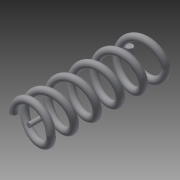
# Autodesk Inventor part: Spring
Saved by Autodesk Inventor 2015 (Build 190159000, 159)
## iProperties
Created: 2017-01-08
Part Number: Spring
Material: Generic
Document SubType Name: Modeling
Designer: Ernest
Density: 1 g/cm^3
Appearance: Default
Mass: 0.268639 g
Surface Area: 7.30223 cm^2
Volume: 0.268639 cm^3
Author: Ernest
Autodesk Inventor part; units mm, degrees
ref_plane "YZ Plane" through (0, 0, 0) normal (1, 0, 0) x (0, 1, 0)
ref_plane "XZ Plane" through (0, 0, 0) normal (0, 1, 0) x (-1, 0, 0)
ref_plane "XY Plane" through (0, 0, 0) normal (0, 0, 1) x (1, 0, 0)
sketch "Sketch1" plane through (0, 0, 0) normal (0, 0, 1) x (1, 0, 0)
  line L0 (0, 0) -> (0, 25)
  circle A0 centre (4, 0) radius 0.75
  dimension "d0" = 25
  dimension "d1" = 1.5
  dimension "d2" = 4
  constraints: 2 end point, 1 centre point, 1 vertical
  measures "d0" distance of L0.start L0.end
  measures "d1" diameter of A0
  measures "d2" distance of L0.start A0.centre
coil "Coil1" sketch "Sketch1" operation add axis through (0, 0, 0) along (0, 1, 0) pitch 5 turns 5 hand right
sketch "Sketch2" plane through (4, 0, 0) normal (0, 0, 1) x (1, 0, 0)
  circle A0 centre (0, 0) radius 0.75
  line L0 (-4, 0) -> (-4, -1.8881)
  constraints: 2 end point, 1 centre point, 1 vertical
revolve "Revolution1" add sketch "Sketch2" angle 180 about axis through (0, 0, 0) along (0, -1, 0)
sketch "Sketch3" plane through (4, 25, 0) normal (0, 0, -1) x (-1, 0, 0)
  circle A0 centre (0, 0) radius 0.75 projected
  line L0 (4, 0) -> (4, 3.1706)
  point P0 (4, -25)
  point P1 (-0.75, 0)
  constraints: 2 end point, 1 horizontal alignment, 1 vertical
revolve "Revolution2" add sketch "Sketch3" angle 180 about axis through (0, 25, 0) along (0, 1, 0)
sketch "Sketch4" plane through (0, 0, 0) normal (0, 1, 0) x (-1, 0, 0)
  circle A0 centre (0, 0) radius 0.5
  dimension "d13" = 1
  constraints: 1 centre point, 1 coincident
  measures "d13" diameter of A0
extrude "Extrusion1" add sketch "Sketch4" along normal blind 2 and the other way blind 0.75
body "Solid1"
